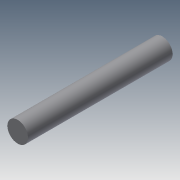
# Autodesk Inventor part: hridelka_packa
Saved by Autodesk Inventor 2013 (Build 170138000, 138)
## iProperties
Created: 2013-05-25
Part Number: hridelka_packa
Material: Generic
Document SubType Name: Modeling
Designer: idle-rug
Density: 1 g/cm^3
Author: idle-rug
Autodesk Inventor part; units mm, degrees
ref_plane "YZ Plane" through (0, 0, 0) normal (1, 0, 0) x (0, 1, 0)
ref_plane "XZ Plane" through (0, 0, 0) normal (0, 1, 0) x (-1, 0, 0)
ref_plane "XY Plane" through (0, 0, 0) normal (0, 0, 1) x (1, 0, 0)
sketch "Sketch1" plane through (0, 0, 0) normal (0, 1, 0) x (-1, 0, 0)
  circle A0 centre (0, 0) radius 2
  dimension "d0" = 4
  constraints: 1 centre point, 1 coincident
  measures "d0" diameter of A0
extrude "Extrusion1" add sketch "Sketch1" along normal blind 28
body "Solid1"
